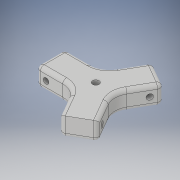
# Autodesk Inventor part: Custom_Delta_End_Effector
Saved by Autodesk Inventor 2019 (Build 230136000, 136)
## iProperties
Created: 2019-07-09
Part Number: Custom_Delta_End_Effector
Material: Generic
Document SubType Name: Modeling
Designer: Jorian Brusind
Density: 1 g/cm^3
Appearance: Default
Author: Jorian Brusind
Autodesk Inventor part; units mm, degrees
ref_plane "YZ Plane" through (0, 0, 0) normal (1, 0, 0) x (0, 1, 0)
ref_plane "XZ Plane" through (0, 0, 0) normal (0, 1, 0) x (-1, 0, 0)
ref_plane "XY Plane" through (0, 0, 0) normal (0, 0, 1) x (1, 0, 0)
sketch "Sketch5" plane through (0, 0, 0) normal (0, 1, 0) x (-1, 0, 0)
  circle A0 centre (0, 0) radius 1.75
  circle A1 centre (0, 0) radius 24
  line L0 (0, 0) -> (24, 0)
  line L1 (24, 0) -> (29, 0)
  line L2 (24, 0) -> (24, -7.5)
  line L3 (24, 0) -> (31.5, 0) construction
  line L4 (24, -7.5) -> (0, -7.5)
  line L5 (0, -7.5) -> (0, 7.5)
  line L6 (0, 7.5) -> (24, 7.5)
  line L7 (24, 7.5) -> (24, -7.5)
  line L8 (-5.5048, 24.5346) -> (6.4952, 3.75)
  line L9 (-6.4952, -3.75) -> (-18.4952, 17.0346)
  line L10 (6.4952, 3.75) -> (-6.4952, -3.75)
  line L11 (-12, 20.7846) -> (-5.5048, 24.5346)
  line L12 (-18.4952, 17.0346) -> (-5.5048, 24.5346)
  line L13 (-18.4952, -17.0346) -> (-6.4952, 3.75)
  line L14 (6.4952, -3.75) -> (-5.5048, -24.5346)
  line L15 (-6.4952, 3.75) -> (6.4952, -3.75)
  line L16 (-12, -20.7846) -> (-18.4952, -17.0346)
  line L17 (-5.5048, -24.5346) -> (-18.4952, -17.0346)
  dimension "d78" = 48
  dimension "d54" = 3.5
  dimension "d82" = 5
  dimension "d83" = 7.5
  dimension "d84" = 90
  dimension "d85" = 24
  dimension "d86" = 15
  dimension "d89" = 360
  constraints: 36 end point, 4 horizontal, 2 coincident, 2 parallel, 2 perpendicular, 2 vertical, 1 centre point, 1 horizontal alignment, 33 other
  measures "d54" diameter of A0
  measures "d82" distance of L0.end L1.end
  measures "d83" distance of L0.end L2.end
  measures "d84" angle of L2 L3
  measures "d85" distance of L5.end L6.end
  measures "d86" distance of L4.end L5.end
extrude "Extrusion7" add sketch "Sketch5" along normal blind 10 contours L0 L10 A0 | L0 A1 L4 L14 L15 A0 | A0 L15 L0 | A0 L10 L8 L6 A1 L0 | L10 L5 A0 | A0 L5 L6 L8 L10 | L15 L14 L4 L5 A0 | A0 L5 L15 | L15 A0 L5 | L5 A0 L10 | L10 A0 L15 | L2 L4 A1 | A1 L6 L7 | A0 L15 L13 L9 A1 L8 L6 L5 | L5 L4 L14 A1 L13 L9 L10 A0 | L10 L9 L13 L15 A0 | A1 L11 L8 | L14 L17 A1 | A1 L9 L12 | L16 L13 A1
sketch "Sketch7" plane through (8.6603, 0, 0) normal (0.8660254, 0, 0.5) x (0.5, 0, -0.8660254)
  line L0 (19.6699, 0) -> (19.6699, 10) projected
  line L1 (19.6699, 10) -> (19.6699, 5)
  line L2 (19.6699, 5) -> (14.6699, 5)
  circle A0 centre (14.6699, 5) radius 1.5
  point P0 (-4.3301, 0)
  dimension "d93" = 5
  dimension "d94" = 5
  dimension "d95" = 3
  constraints: 4 end point, 1 centre point, 1 coincident, 1 midpoint, 1 perpendicular
  measures "d93" distance of L0.end L1.end
  measures "d94" distance of L1.end L2.end
  measures "d95" diameter of A0
extrude "Extrusion8" cut sketch "Sketch7" against normal blind 20
sketch "Sketch8" plane through (0, 10, 0) normal (0, 1, 0) x (1, 0, 0)
  circle A0 centre (0, 0) radius 1.75
  dimension "d98" = 3.5
  constraints: 1 centre point, 1 coincident
  measures "d98" diameter of A0
extrude "Extrusion9" cut sketch "Sketch8" against normal blind 10
pattern_circular "Circular Pattern7" count 3 over 360 about axis through (0, 10, 0) along (0, -1, 0) of "Extrusion8"
fillet "Fillet7" radius 10 3 edges at (8.6603, 5, 0) (-4.3301, 5, 7.5) (-4.3301, 5, -7.5)
fillet "Fillet8" radius 2 29 edges at (5.5048, 5, 24.5346) (18.4952, 5, 17.0346) (-24, 5, 7.5) (-24, 10, 0) (18.4952, 5, -17.0346) (12, 10, -20.7846) (5.5048, 5, -24.5346) (-5.1036, 10, -8.8397) (-17.0518, 10, -7.5) (2.0307, 10, -18.5173) (15.0211, 10, 11.0173) (15.0211, 10, -11.0173) (10.2073, 10, 0) (-17.0518, 10, 7.5) (2.0307, 10, 18.5173) (-5.1036, 10, 8.8397) (-24, 5, -7.5) (-24, 0, 0) (12, 0, 20.7846) (10.2073, 0, 0) (15.0211, 0, -11.0173) (15.0211, 0, 11.0173) (-5.1036, 0, 8.8397) (-17.0518, 0, 7.5) (2.0307, 0, 18.5173) (-17.0518, 0, -7.5) (2.0307, 0, -18.5173) (-5.1036, 0, -8.8397) (12, 0, -20.7846)
body "Solid3"
